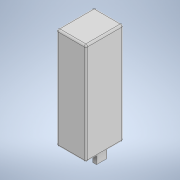
# Autodesk Inventor part: battery2500
Saved by Autodesk Inventor 2020 (Build 240168000, 168)
## iProperties
Created: 2020-01-03
Part Number: battery2500
Material: Generic
Document SubType Name: Modeling
Designer: my
Density: 1 g/cm^3
Appearance: Default
Author: my
Autodesk Inventor part; units mm, degrees
ref_plane "YZ Plane" through (0, 0, 0) normal (1, 0, 0) x (0, 1, 0)
ref_plane "XZ Plane" through (0, 0, 0) normal (0, 1, 0) x (-1, 0, 0)
ref_plane "XY Plane" through (0, 0, 0) normal (0, 0, 1) x (1, 0, 0)
sketch "Sketch1" plane through (0, 0, 0) normal (0, 0, 1) x (1, 0, 0)
  line L0 (0, 0) -> (33.5, 0)
  line L1 (33.5, 0) -> (33.5, -115)
  line L2 (33.5, -115) -> (0, -115)
  line L3 (0, -115) -> (0, 0)
  dimension "d0" = 115
  dimension "d1" = 33.5
  constraints: 8 end point, 2 parallel, 1 horizontal, 1 perpendicular
  measures "d0" distance of L0.end L1.end
  measures "d1" distance of L1.end L2.end
extrude "Extrusion1" add sketch "Sketch1" along normal blind 43
fillet "Fillet1" radius 2 12 edges at (33.5, -57.5, 0) (33.5, 0, 21.5) (33.5, -57.5, 43) (33.5, -115, 21.5) (16.75, -115, 0) (16.75, -115, 43) (0, -115, 21.5) (0, -57.5, 0) (0, -57.5, 43) (0, 0, 21.5) (16.75, 0, 0) (16.75, 0, 43)
sketch "Sketch2" plane through (2, -115, 41) normal (0, -1, 0) x (1, 0, 0)
  line L0 (0, -39) -> (0, 0) projected
  line L1 (0, -26.5048) -> (8.8714, -26.5048)
  line L2 (8.8714, -26.5048) -> (8.8714, -12.339)
  line L3 (8.8714, -12.339) -> (0, -12.339)
  line L4 (0, -12.339) -> (0, -26.5048)
  line L5 (25.0138, -23.8693) -> (29.2965, -23.8693)
  line L6 (29.2965, -23.8693) -> (29.2965, -12.339)
  line L7 (29.2965, -12.339) -> (25.0138, -12.339)
  line L8 (25.0138, -12.339) -> (25.0138, -23.8693)
  point P0 (-2, -41)
  point P1 (0, -12.339)
  constraints: 16 end point, 4 parallel, 2 horizontal, 2 perpendicular, 2 point on line
extrude "Extrusion2" add sketch "Sketch2" along normal blind 10
body "Solid1"
